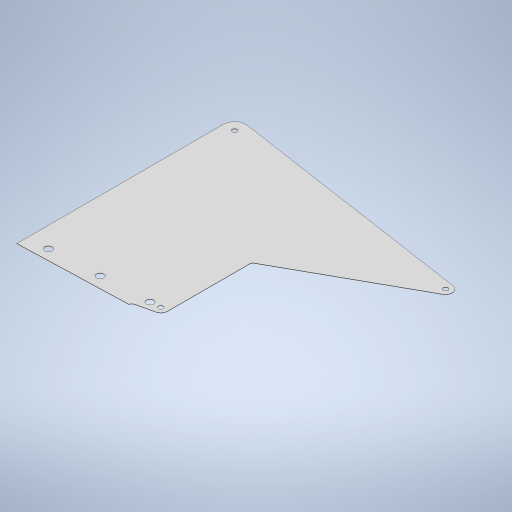
# Autodesk Inventor part: base_main_pcb_p2_itr2
Saved by Autodesk Inventor 2024 (Build 280153000, 153)
## iProperties
Created: 2026-03-21
Part Number: base_main_pcb_p2_itr2
Material: Generic
Document SubType Name: Modeling
Designer: schar
Density: 1 g/cm^3
Appearance: Default
Author: schar
Autodesk Inventor part; units mm, degrees
ref_plane "YZ Plane" through (0, 0, 0) normal (1, 0, 0) x (0, 1, 0)
ref_plane "XZ Plane" through (0, 0, 0) normal (0, 1, 0) x (-1, 0, 0)
ref_plane "Work Plane1" through (-203, 0.6, 290) normal (0, 1, 0) x (1, 0, 0)
sketch "Sketch1" plane through (-203, 0.6, 290) normal (0, 1, 0) x (1, 0, 0)
  line L0 (-2, 272.9952) -> (-2, 2) projected
  arc A0 (73.455, 136.4093) -> (71.909, 134.5363) centre (73.9075, 134.4612) ccw projected
  line L1 (-2, 132.2079) -> (71.909, 134.5363)
  arc A1 (84.5, 138.975) -> (89, 143.475) centre (84.5, 143.475) ccw projected
  arc A2 (84.5, 138.975) -> (89, 143.475) centre (84.5, 143.475) ccw projected
  arc A3 (84.5, 138.975) -> (89, 143.475) centre (84.5, 143.475) ccw projected
  line L2 (73.455, 136.4093) -> (84.5, 138.975) projected
  line L3 (73.455, 136.4093) -> (84.5, 138.975) projected
  line L4 (73.455, 136.4093) -> (84.5, 138.975) projected
  line L5 (73.455, 136.4093) -> (84.5, 138.975) projected
  line L6 (89, 143.475) -> (89, 199.525) projected
  line L7 (89, 143.475) -> (89, 199.525) projected
  line L8 (89, 143.475) -> (89, 199.525) projected
  line L9 (89, 143.475) -> (89, 199.525) projected
  arc A4 (90.0288, 201.2733) -> (89, 199.525) centre (91, 199.525) ccw projected
  arc A5 (90.0288, 201.2733) -> (89, 199.525) centre (91, 199.525) ccw projected
  arc A6 (90.0288, 201.2733) -> (89, 199.525) centre (91, 199.525) ccw projected
  line L10 (90.0288, 201.2733) -> (172.6853, 247.1912) projected
  line L11 (90.0288, 201.2733) -> (172.6853, 247.1912) projected
  line L12 (90.0288, 201.2733) -> (172.6853, 247.1912) projected
  line L13 (90.0288, 201.2733) -> (172.6853, 247.1912) projected
  arc A7 (6.6087, 280.0995) -> (-2, 272.9952) centre (5.5, 272.675) ccw projected
  line L14 (170.5, 255.625) -> (6.6087, 280.0995) projected
  line L15 (170.5, 255.625) -> (6.6087, 280.0995) projected
  line L16 (170.5, 255.625) -> (6.6087, 280.0995) projected
  line L17 (170.5, 255.625) -> (6.6087, 280.0995) projected
  circle A8 centre (5.5, 272.675) radius 1.675 projected
  circle A9 centre (170.5, 251.125) radius 1.675 projected
  arc A10 (172.6853, 247.1912) -> (170.5, 255.625) centre (170.5, 251.125) ccw projected
  arc A11 (172.6853, 247.1912) -> (170.5, 255.625) centre (170.5, 251.125) ccw projected
  circle A12 centre (170.5, 251.125) radius 1.675 projected
  circle A13 centre (84.5, 143.475) radius 1.675 projected
  circle A14 centre (84.5, 143.475) radius 1.675 projected
  circle A15 centre (84.5, 143.475) radius 1.675 projected
  circle A16 centre (84.5, 143.475) radius 1.675 projected
  arc A17 (73.455, 136.4093) -> (71.909, 134.5363) centre (73.9075, 134.4612) ccw projected
  arc A18 (73.455, 136.4093) -> (71.909, 134.5363) centre (73.9075, 134.4612) ccw projected
  arc A19 (90.0288, 201.2733) -> (89, 199.525) centre (91, 199.525) ccw projected
  arc A20 (84.5, 138.975) -> (89, 143.475) centre (84.5, 143.475) ccw projected
  arc A21 (73.455, 136.4093) -> (71.909, 134.5363) centre (73.9075, 134.4612) ccw projected
  circle A22 centre (5.5, 272.675) radius 1.675 projected
  circle A23 centre (5.5, 272.675) radius 1.675 projected
  circle A24 centre (5.5, 272.675) radius 1.675 projected
  arc A25 (6.6087, 280.0995) -> (-2, 272.9952) centre (5.5, 272.675) ccw projected
  arc A26 (6.6087, 280.0995) -> (-2, 272.9952) centre (5.5, 272.675) ccw projected
  arc A27 (6.6087, 280.0995) -> (-2, 272.9952) centre (5.5, 272.675) ccw projected
  circle A28 centre (170.5, 251.125) radius 1.675 projected
  circle A29 centre (170.5, 251.125) radius 1.675 projected
  arc A30 (172.6853, 247.1912) -> (170.5, 255.625) centre (170.5, 251.125) ccw projected
  arc A31 (172.6853, 247.1912) -> (170.5, 255.625) centre (170.5, 251.125) ccw projected
  line L18 (89, 148.562) -> (-2, 148.562) projected
  line L19 (89, 148.562) -> (-2, 148.562) projected
  arc A32 (73.455, 136.4093) -> (71.909, 134.5363) centre (73.9075, 134.4612) ccw projected
  arc A33 (73.455, 136.4093) -> (71.909, 134.5363) centre (73.9075, 134.4612) ccw projected
  line L20 (73.455, 136.4093) -> (84.5, 138.975) projected
  line L21 (73.455, 136.4093) -> (84.5, 138.975) projected
  arc A34 (84.5, 138.975) -> (89, 143.475) centre (84.5, 143.475) ccw projected
  line L22 (73.455, 136.4093) -> (84.5, 138.975) projected
  line L23 (73.455, 136.4093) -> (84.5, 138.975) projected
  arc A35 (84.5, 138.975) -> (89, 143.475) centre (84.5, 143.475) ccw projected
  arc A36 (84.5, 138.975) -> (89, 143.475) centre (84.5, 143.475) ccw projected
  arc A37 (84.5, 138.975) -> (89, 143.475) centre (84.5, 143.475) ccw projected
  circle A38 centre (84.5, 143.475) radius 1.675 projected
  circle A39 centre (84.5, 143.475) radius 1.675 projected
  circle A40 centre (84.5, 143.475) radius 1.675 projected
  circle A41 centre (77.6916, 142.9267) radius 2.5 projected
  circle A42 centre (77.6916, 142.9267) radius 2.5 projected
  circle A43 centre (77.6916, 142.9267) radius 2.5 projected
  circle A44 centre (45.3956, 141.3608) radius 2.5 projected
  circle A45 centre (45.3956, 141.3608) radius 2.5 projected
  circle A46 centre (45.3956, 141.3608) radius 2.5 projected
  circle A47 centre (45.3956, 141.3608) radius 2.5 projected
  circle A48 centre (45.3956, 141.3608) radius 2.5 projected
  circle A49 centre (11.7945, 139.7317) radius 2.5 projected
  circle A50 centre (11.7945, 139.7317) radius 2.5 projected
  circle A51 centre (11.7945, 139.7317) radius 2.5 projected
  circle A52 centre (11.7945, 139.7317) radius 2.5 projected
  circle A53 centre (11.7945, 139.7317) radius 2.5 projected
  line L24 (89, 148.562) -> (-2, 148.562) projected
  line L25 (89, 148.562) -> (-2, 148.562) projected
  arc A54 (73.455, 136.4093) -> (71.909, 134.5363) centre (73.9075, 134.4612) ccw projected
  arc A55 (73.455, 136.4093) -> (71.909, 134.5363) centre (73.9075, 134.4612) ccw projected
  circle A56 centre (77.6916, 142.9267) radius 2.5 projected
  circle A57 centre (77.6916, 142.9267) radius 2.5 projected
  line L26 (89, 143.475) -> (89, 148.562) projected
  line L27 (89, 143.475) -> (89, 148.562) projected
  line L28 (89, 143.475) -> (89, 148.562) projected
  line L29 (89, 143.475) -> (89, 148.562) projected
  circle A58 centre (84.5, 143.475) radius 1.675 projected
  point P0 (203, 290)
  constraints: 2 end point, 1 point on line, 8 other
extrude "Extrusion1" add sketch "Sketch1" along normal blind 0.2
body "Solid2"
